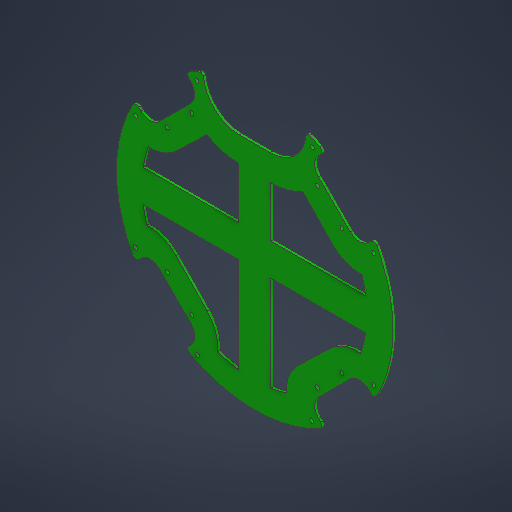
# Autodesk Inventor part: Boden WM
Saved by Autodesk Inventor 2025.3 (Build 293356000, 356)
## iProperties
Created: 2025-07-13
Part Number: Boden WM
Material: Generisch
Document SubType Name: Modeling
Designer: theod
Density: 1 g/cm^3
Appearance: Vorgabe
Author: theod
Autodesk Inventor part; units mm, degrees
ref_plane "YZ Plane" through (0, 0, 0) normal (1, 0, 0) x (0, 1, 0)
ref_plane "XZ Plane" through (0, 0, 0) normal (0, 1, 0) x (-1, 0, 0)
ref_plane "XY Plane" through (0, 0, 0) normal (0, 0, 1) x (1, 0, 0)
sketch "Skizze1" plane through (0, 0, 0) normal (0, 1, 0) x (-1, 0, 0)
  circle A0 centre (-44.3776, -92.6293) radius 1.6
  circle A1 centre (92.6293, 44.3776) radius 1.6
  circle A2 centre (-92.6293, -44.3776) radius 1.6
  circle A3 centre (44.3776, -92.6293) radius 1.6
  circle A4 centre (92.6293, -44.3776) radius 1.6
  circle A5 centre (-92.6293, 44.3776) radius 1.6
  circle A6 centre (45, 91.781) radius 1.6
  circle A7 centre (-45, 91.781) radius 1.6
  arc A8 (12, 71.7738) -> (39.8653, 97.0306) centre (12, 99.7738) ccw
  line L0 (-12, 71.7738) -> (12, 71.7738)
  arc A9 (-39.8653, 97.0306) -> (-12, 71.7738) centre (-12, 99.7738) ccw
  arc A10 (-39.8653, 97.0306) -> (-42.6492, 98.6705) centre (-41.8557, 96.8347) ccw
  arc A11 (-42.6492, 98.6705) -> (-50.5184, 94.8829) centre (0, -0.0072) ccw
  arc A12 (-50.5184, 94.8829) -> (-51.2299, 90.1135) centre (-49.1086, 92.2348) ccw
  line L1 (-49.4975, 88.3811) -> (-51.2299, 90.1135)
  arc A13 (-49.4975, 74.239) -> (-49.4975, 88.3811) centre (-56.5685, 81.31) ccw
  line L2 (-74.2462, 49.4902) -> (-49.4975, 74.239)
  arc A14 (-88.3883, 49.4902) -> (-74.2462, 49.4902) centre (-81.3173, 56.5613) ccw
  line L3 (-90.1208, 51.2226) -> (-88.3883, 49.4902)
  arc A15 (-90.1208, 51.2226) -> (-94.8902, 50.5111) centre (-92.2421, 49.1013) ccw
  arc A16 (-94.8902, 50.5111) -> (-94.8902, -50.5256) centre (0, -0.0072) ccw
  arc A17 (-94.8902, -50.5256) -> (-90.1207, -51.2371) centre (-92.2421, -49.1158) ccw
  line L4 (-88.3883, -49.5047) -> (-90.1207, -51.2371)
  arc A18 (-74.2462, -49.5047) -> (-88.3883, -49.5047) centre (-81.3173, -56.5758) ccw
  line L5 (-49.4975, -74.2535) -> (-74.2462, -49.5047)
  arc A19 (-49.4975, -88.3956) -> (-49.4975, -74.2535) centre (-56.5685, -81.3245) ccw
  line L6 (-51.2299, -90.128) -> (-49.4975, -88.3956)
  arc A20 (-51.2299, -90.128) -> (-50.5184, -94.8974) centre (-49.1086, -92.2493) ccw
  arc A21 (-50.5184, -94.8974) -> (50.5184, -94.8974) centre (0, -0.0072) ccw
  arc A22 (50.5184, -94.8974) -> (51.2299, -90.128) centre (49.1086, -92.2493) ccw
  line L7 (49.4975, -88.3956) -> (51.2299, -90.128)
  arc A23 (49.4975, -74.2535) -> (49.4975, -88.3956) centre (56.5685, -81.3245) ccw
  line L8 (74.2462, -49.5047) -> (49.4975, -74.2535)
  arc A24 (88.3883, -49.5047) -> (74.2462, -49.5047) centre (81.3173, -56.5758) ccw
  line L9 (90.1208, -51.2371) -> (88.3883, -49.5047)
  arc A25 (90.1208, -51.2371) -> (94.8902, -50.5256) centre (92.2421, -49.1158) ccw
  arc A26 (94.8902, -50.5256) -> (94.8902, 50.5111) centre (0, -0.0072) ccw
  arc A27 (94.8902, 50.5111) -> (90.1207, 51.2226) centre (92.2421, 49.1013) ccw
  line L10 (88.3883, 49.4902) -> (90.1207, 51.2226)
  arc A28 (74.2462, 49.4902) -> (88.3883, 49.4902) centre (81.3173, 56.5613) ccw
  line L11 (49.4975, 74.239) -> (74.2462, 49.4902)
  arc A29 (49.4975, 88.3811) -> (49.4975, 74.239) centre (56.5685, 81.31) ccw
  line L12 (51.2299, 90.1135) -> (49.4975, 88.3811)
  arc A30 (51.2299, 90.1135) -> (50.5184, 94.8829) centre (49.1086, 92.2348) ccw
  arc A31 (50.5184, 94.8829) -> (42.6492, 98.6705) centre (0, -0.0072) ccw
  arc A32 (42.6492, 98.6705) -> (39.8653, 97.0306) centre (41.8557, 96.8347) ccw
  circle A33 centre (-48.7904, 67.8822) radius 1.6
  circle A34 centre (48.7904, 67.8823) radius 1.6
  circle A35 centre (67.8822, 48.7904) radius 1.6
  circle A36 centre (-67.8823, 48.7904) radius 1.6
  circle A37 centre (67.8823, -48.7904) radius 1.6
  circle A38 centre (48.7904, -67.8822) radius 1.6
  circle A39 centre (-48.7904, -67.8823) radius 1.6
  circle A40 centre (-67.8822, -48.7904) radius 1.6
  arc A41 (-83.3481, 25.2693) -> (-60.278, 34.4345) centre (-81.8968, 55.2341) ccw
  arc A42 (-58.8889, -36.4356) -> (-82.2957, -28.1679) centre (-79.6885, -58.0544) ccw
  line L13 (-58.8889, -36.4356) -> (-49.1604, -45.7954)
  line L14 (-49.1604, -45.7954) -> (-43.3954, -51.342)
  line L15 (-43.3954, -51.342) -> (-33.6669, -60.7018)
  arc A43 (-24.5017, -83.772) -> (-33.6669, -60.7018) centre (-54.4666, -82.3207) ccw
  arc A44 (37.0306, -59.3366) -> (28.7629, -82.7434) centre (58.6494, -80.1363) ccw
  line L16 (37.0306, -59.3366) -> (46.3904, -49.6081)
  line L17 (46.3904, -49.6081) -> (51.937, -43.8431)
  line L18 (51.937, -43.8431) -> (61.2969, -34.1146)
  arc A45 (83.8457, -25.0231) -> (61.2969, -34.1146) centre (82.8273, -55.0058) ccw
  arc A46 (60.905, 36.457) -> (82.8171, 28.2415) centre (81.5589, 58.2151) ccw
  line L19 (60.905, 36.457) -> (51.1766, 45.8169)
  line L20 (51.1766, 45.8169) -> (45.4116, 51.3634)
  line L21 (45.4116, 51.3634) -> (37.2169, 59.4013)
  arc A47 (12.5, 52.2686) -> (37.2169, 59.4013) centre (12.0366, 100.2664) ccw
  line L22 (-12.47, 51.7864) -> (-12.5, 51.7858)
  arc A48 (-37.4131, 58.1998) -> (-12.5, 51.7858) centre (-13.4268, 99.7769) ccw
  line L23 (-37.4131, 58.1998) -> (-45.3715, 49.9279)
  line L24 (-45.3715, 49.9279) -> (-50.9181, 44.1629)
  line L25 (-50.9181, 44.1629) -> (-60.278, 34.4345)
  line L26 (12.5, 12.4928) -> (12.5, 52.2686)
  line L27 (-12.5, 12.4928) -> (-12.5, 51.7858)
  line L28 (12.5, -12.5072) -> (86.6015, -12.5072)
  line L29 (12.5, 12.4928) -> (86.6036, 12.4928)
  line L30 (12.5, -12.5072) -> (12.5, -86.6025)
  line L31 (-12.5, -12.5072) -> (-12.5, -86.452)
  line L32 (-12.5, -12.5072) -> (-86.0925, -12.5072)
  line L33 (-12.4928, 12.4928) -> (-86.1498, 12.4928)
  arc A49 (-83.3481, 25.2693) -> (-86.1498, 12.4928) centre (0.4811, 0.1913) ccw
  arc A50 (-86.0925, -12.5072) -> (-82.2957, -28.1679) centre (0.4811, 0.1913) ccw
  arc A51 (83.8457, -25.0231) -> (86.6015, -12.5072) centre (0, 0) ccw
  arc A52 (86.6036, 12.4928) -> (82.8171, 28.2415) centre (0, 0) ccw
  arc A53 (-24.5017, -83.772) -> (-12.5, -86.452) centre (0.5214, 0.0737) ccw
  arc A54 (12.5, -86.6025) -> (28.7629, -82.7434) centre (0.5214, 0.0737) ccw
  constraints: 78 point on circle, 68 end point, 55 centre point, 3 parallel, 3 perpendicular, 3 point on line, 1 vertical
extrude "Extrusion1" add sketch "Skizze1" along normal blind 2
